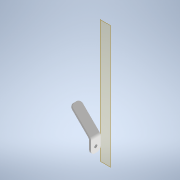
# Autodesk Inventor part: 30_Cameraholder
Saved by Autodesk Inventor 2022 (Build 260153000, 153)
## iProperties
Created: 2022-06-16
Part Number: 30_Cameraholder
Material: Generisch
Document SubType Name: Modeling
Designer: diederichbenedict
Density: 1 g/cm^3
Appearance: Vorgabe
Author: diederichbenedict
Autodesk Inventor part; units mm, degrees
ref_plane "YZ Plane" through (0, 0, 0) normal (1, 0, 0) x (0, 1, 0)
ref_plane "XZ Plane" through (0, 0, 0) normal (0, 1, 0) x (-1, 0, 0)
ref_plane "XY Plane" through (0, 0, 0) normal (0, 0, 1) x (1, 0, 0)
ref_plane "Arbeitsebene1" through (0, 0, 0) normal (0, 0, 1) x (1, 0, 0)
sketch "Skizze1" plane through (0, 0, 0) normal (0, 0, 1) x (1, 0, 0)
  line L0 (0, 10.5) -> (-10, 10.5)
  line L1 (0, 13.3) -> (-10, 13.3)
  line L2 (-10, 0) -> (-10, 117.8) projected
  line L3 (-10, 4.5) -> (-12, 4.5)
  line L4 (-12, 4.5) -> (-12, 19.5)
  line L5 (-12, 19.5) -> (-10, 19.5)
  line L6 (-10, 19.5) -> (-10, 4.5)
  line L7 (-10, 19.5) -> (-31.2883, 40.6378)
  line L8 (-31.2883, 40.6378) -> (-32.6975, 39.2186)
  line L9 (-32.6975, 39.2186) -> (-12, 18.6674)
  line L10 (-28.996, 38.3616) -> (-8.6029, 58.9) construction
  line L11 (2, 58.9) -> (-12, 58.9)
  point P0 (0, 0)
  dimension "d0" = 2
  dimension "d1" = 15
  dimension "d2" = 6
  dimension "d3" = 2
  dimension "d4" = 30
  dimension "d5" = 90
  constraints: 22 end point, 4 horizontal, 4 point on line, 3 perpendicular, 2 parallel, 6 other
  measures "d0" distance of L4.end L5.end
  measures "d1" distance of L3.end L4.end
  measures "d2" distance between parallel lines of L0 L3
  measures "d3" distance of L7.end L8.end
  measures "d4" distance from line of L8 L5.end
  measures "d5" angle of L10 L7
extrude "Extrusion1" add sketch "Skizze1" along normal blind 10
fillet "Rundung1" radius 4 6 edges at (-12, 18.6674, 5) (-10, 19.5, 5) (-11, 4.5, 10) (-11, 4.5, 0) (-31.9929, 39.9282, 10) (-31.9929, 39.9282, 0)
sketch "Skizze2" plane through (-12, 8.5, 0) normal (-1, 0, 0) x (0, 0, 1)
  arc A0 (0, 0) -> (4, -4) centre (4, 0) ccw projected
  line L0 (4, -4) -> (6, -4) projected
  arc A1 (6, -4) -> (10, 0) centre (6, 0) ccw projected
  line L1 (10, 8.5022) -> (10, 0) projected
  line L2 (0, 8.5022) -> (10, 8.5022) projected
  line L3 (0, 8.5022) -> (0, 0) projected
  circle A2 centre (5, 2) radius 1.6
  point P0 (0, -8.5)
  dimension "d9" = 3.2
  dimension "d10" = 6
  constraints: 1 centre point
  measures "d9" diameter of A2
  measures "d10" distance from line of A2.centre L0
extrude "Extrusion2" cut sketch "Skizze2" against normal blind 10 contours A2
